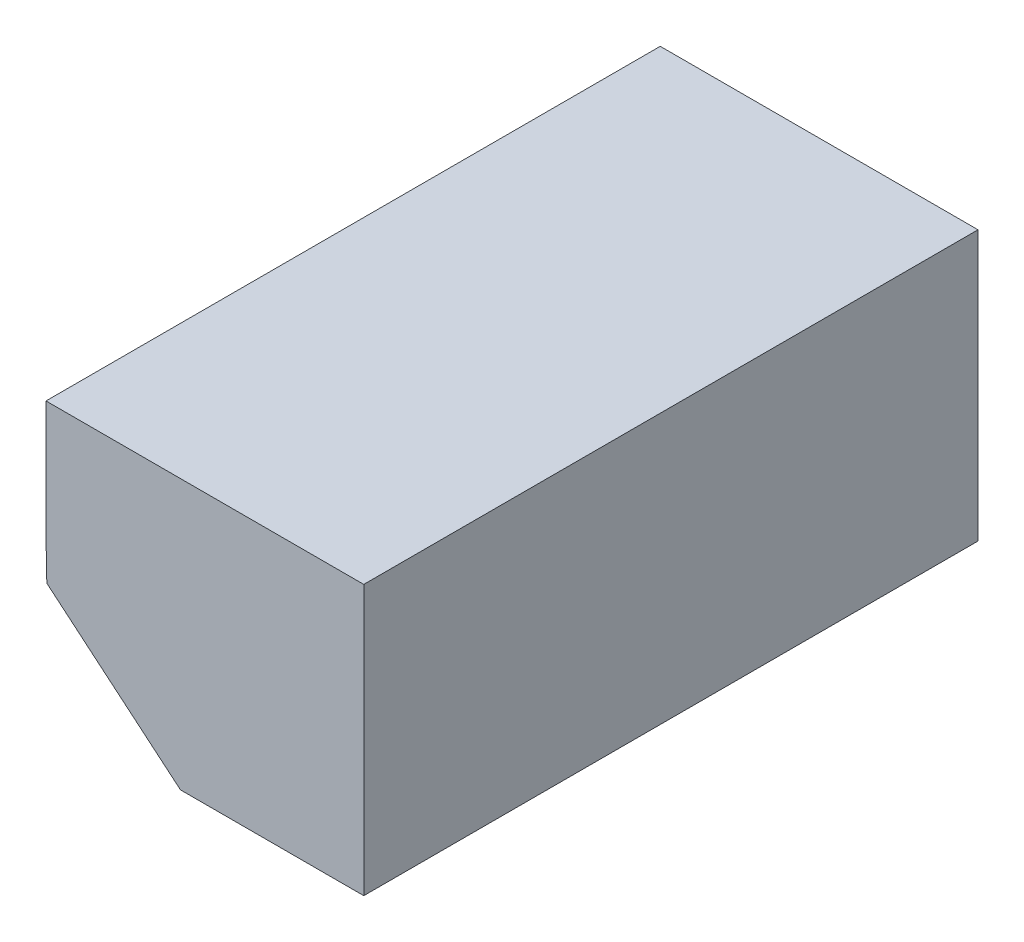
# Autodesk Inventor part: DUMMY 3
Saved by Autodesk Inventor 2024.2 (Build 282272000, 272)
## iProperties
Created: 2024-06-16
Part Number: DUMMY 3
Material: Generic
Document SubType Name: Modeling
Designer: admin
Density: 1 g/cm^3
Appearance: Default
Author: admin
Autodesk Inventor part; units mm, degrees
ref_plane "YZ Plane" through (0, 0, 0) normal (1, 0, 0) x (0, 1, 0)
ref_plane "XZ Plane" through (0, 0, 0) normal (0, 1, 0) x (-1, 0, 0)
ref_plane "XY Plane" through (0, 0, 0) normal (0, 0, 1) x (1, 0, 0)
sketch "Sketch1" plane through (0, 0, 0) normal (0, 0, 1) x (1, 0, 0)
  line L0 (-7604.7986, 5796.6031) -> (-7604.7986, 5308.6026) projected
  line L1 (-6828.8058, 5566.6031) -> (-6828.8058, 5596.6031) projected
  line L2 (-7276.4637, 4938.2305) -> (-7602.7986, 5212.058) projected
  line L3 (-6828.8058, 5596.6031) -> (-7604.7986, 5596.6031)
  line L4 (-7604.7986, 5308.6026) -> (-7602.7986, 5212.058)
  line L5 (-6828.8058, 5566.6031) -> (-6828.8058, 4938.2305)
  line L6 (-6828.8058, 4938.2305) -> (-7276.4637, 4938.2305)
  point P0 (0, 0)
  constraints: 8 end point, 2 perpendicular, 1 point on line, 1 vertical
extrude "Extrusion1" add sketch "Sketch1" along normal mid plane 1500
body "Solid1"
